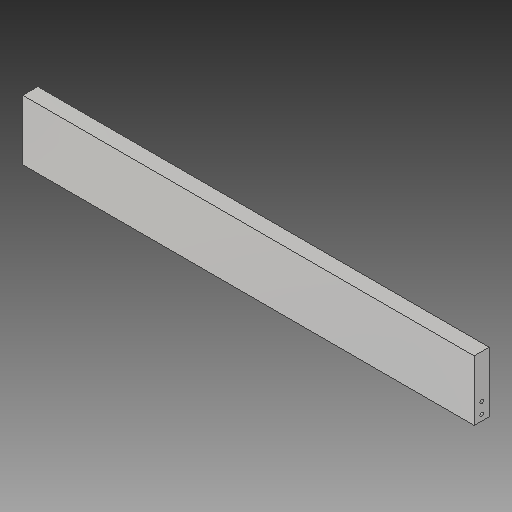
# Autodesk Inventor part: Xcolum
Saved by Autodesk Inventor 2019 (Build 230136000, 136)
## iProperties
Created: 2018-10-03
Part Number: Xcolum
Material: Aluminum 6061-AHC
Document SubType Name: Modeling
Designer: LillaHunden
Mass: 324 g
Surface Area: 308 cm^2
Volume: 120 cm^3
Density: 2.7 g/cm^3
Appearance: Aluminum - Dark
Author: LillaHunden
Autodesk Inventor part; units mm, degrees
ref_plane "YZ Plane" through (0, 0, 0) normal (1, 0, 0) x (0, 1, 0)
ref_plane "XZ Plane" through (0, 0, 0) normal (0, 1, 0) x (-1, 0, 0)
ref_plane "XY Plane" through (0, 0, 0) normal (0, 0, 1) x (1, 0, 0)
sketch "Sketch1" plane through (0, 0, 0) normal (0, 0, 1) x (1, 0, 0)
  line L0 (0, -29.1453) -> (300, -29.1453)
  line L1 (300, -29.1453) -> (300, 10.8547)
  line L2 (300, 10.8547) -> (0, 10.8547)
  line L3 (0, 10.8547) -> (0, -29.1453)
  point P0 (0, 0)
  dimension "d0" = 300
  dimension "d1" = 40
  constraints: 8 end point, 2 parallel, 1 horizontal, 1 perpendicular
  measures "d0" distance of L2.end L1.end
  measures "d1" distance of L1.end L0.end
extrude "Extrusion1" add sketch "Sketch1" along normal blind 10
sketch "Sketch2" plane through (300, -29.1453, 0) normal (1, 0, 0) x (0, 0, -1)
  point P0 (-5, 3.8516)
  point P1 (-5, 11.1484)
  point P2 (4.1697, 3.85)
  point P3 (4.1697, 11.15)
hole "Hole1" at (300, -25.2937, 5) at (300, -17.9969, 5) at (300, -25.2953, -4.1697) at (300, -17.9953, -4.1697) direction (-1, 0, 0) diameter 2.459 depth 11.1 tip angle 120 thread size "M3x0.5" class "6H" standard "ISO Metric profile"
body "Solid1"
